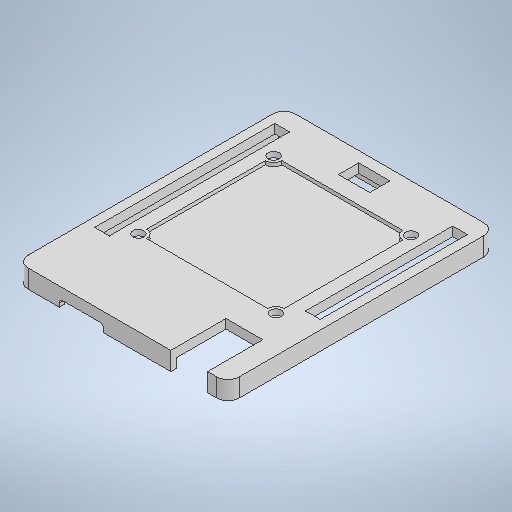
# Autodesk Inventor part: uno_r4_lid
Saved by Autodesk Inventor 2025.2 (Build 292293000, 293)
## iProperties
Created: 2025-03-24
Part Number: uno_r4_lid
Material: Generic
Document SubType Name: Modeling
Designer: caomi
Density: 1 g/cm^3
Appearance: Default
Author: caomi
Autodesk Inventor part; units mm, degrees
ref_plane "YZ Plane" through (0, 0, 0) normal (1, 0, 0) x (0, 1, 0)
ref_plane "XZ Plane" through (0, 0, 0) normal (0, 1, 0) x (-1, 0, 0)
ref_plane "XY Plane" through (0, 0, 0) normal (0, 0, 1) x (1, 0, 0)
sketch "Sketch1" plane through (0, 0, 0) normal (0, 1, 0) x (-1, 0, 0)
  line L0 (0, 0) -> (53.34, 0) construction
  line L1 (53.34, 0) -> (53.34, -68.58) construction
  line L2 (53.34, -68.58) -> (0, -68.58) construction
  line L3 (0, -68.58) -> (0, 0) construction
  line L4 (55.34, -70.58) -> (55.34, 2)
  line L5 (55.34, 2) -> (-2, 2)
  line L6 (-2, 2) -> (-2, -70.58)
  line L7 (-2, -70.58) -> (55.34, -70.58)
  dimension "d0" = 53.34
  dimension "d1" = 68.58
  dimension "d2" = 2
  constraints: 16 end point, 4 parallel, 2 perpendicular, 1 horizontal, 3 other
  measures "d0" distance of L0.start L0.end
  measures "d1" distance of L2.end L0.start
  measures "d2" distance between parallel lines of L1 L4
extrude "Extrusion1" add sketch "Sketch1" against normal blind 5
fillet "Fillet1" radius 3 4 edges at (-55.34, -2.5, 2) (-55.34, -2.5, -70.58) (2, -2.5, -70.58) (2, -2.5, 2)
shell "Shell1" thickness 1.5 removed faces 1 at (-17.1133, -5, -45.3867)
sketch "Sketch2" plane through (0, -5, 0) normal (0, -1, 0) x (1, 0, 0)
  line L0 (-53.34, 0) -> (-53.34, -68.58) construction
  line L1 (-52.34, 0.5) -> (-1, 0.5) projected
  line L2 (-1, 2) -> (-52.34, 2) projected
  line L3 (-43.84, 0.5) -> (-31.84, 0.5)
  line L4 (-31.84, 0.5) -> (-31.84, 2)
  line L5 (-31.84, 2) -> (-43.84, 2)
  line L6 (-43.84, 2) -> (-43.84, 0.5)
  line L7 (-13.54, 2) -> (-3.54, 2)
  line L8 (-3.54, 2) -> (-3.54, -13)
  line L9 (-3.54, -13) -> (-13.54, -13)
  line L10 (-13.54, -13) -> (-13.54, 2)
  dimension "d8" = 12
  dimension "d15" = 9.5
  dimension "d16" = 39.8
  dimension "d17" = 10
  dimension "d18" = 15
  constraints: 16 end point, 4 parallel, 3 point on line, 2 horizontal, 2 perpendicular
  measures "d8" distance between parallel lines of L4 L6
  measures "d15" distance from line of L0 L5.end
  measures "d16" distance between parallel lines of L0 L10
  measures "d17" distance between parallel lines of L8 L10
  measures "d18" distance of L9.end L7.start
extrude "Extrusion2" cut sketch "Sketch2" against normal blind 2 contours L6 L2 L4 L1
fillet "Fillet2" radius 1 2 edges at (-43.84, -3, 1.25) (-31.84, -3, 1.25)
extrude "Extrusion3" cut sketch "Sketch2" against normal through all contours L10 L2 L8 L1 | L1 L8 L9 L10
sketch "Sketch3" plane through (0, 0, 0) normal (0, 1, 0) x (1, 0, 0)
  line L0 (-53.34, 0) -> (-53.34, 68.58) construction
  line L1 (-52.84, 65.58) -> (-48.84, 65.58)
  line L2 (-48.84, 65.58) -> (-48.84, 16.58)
  line L3 (-48.84, 16.58) -> (-52.84, 16.58)
  line L4 (-52.84, 16.58) -> (-52.84, 65.58)
  line L5 (-53.34, 68.58) -> (0, 68.58) construction
  line L6 (-0.5, 65.58) -> (-4.5, 65.58)
  line L7 (-4.5, 65.58) -> (-4.5, 25.58)
  line L8 (-4.5, 25.58) -> (-0.5, 25.58)
  line L9 (-0.5, 25.58) -> (-0.5, 65.58)
  line L10 (0, 68.58) -> (0, 0) construction
  line L11 (-32.14, 67.68) -> (-23.64, 67.68)
  line L12 (-23.64, 67.68) -> (-23.64, 62.18)
  line L13 (-23.64, 62.18) -> (-32.14, 62.18)
  line L14 (-32.14, 62.18) -> (-32.14, 67.68)
  dimension "d19" = 0.5
  dimension "d20" = 4
  dimension "d23" = 3
  dimension "d24" = 52
  dimension "d25" = 0.5
  dimension "d26" = 3
  dimension "d27" = 40
  dimension "d28" = 21.2
  dimension "d29" = 8.5
  dimension "d30" = 5.5
  dimension "d31" = 0.9
  constraints: 24 end point, 6 parallel, 3 horizontal, 3 perpendicular, 1 collinear
  measures "d19" distance between parallel lines of L0 L4
  measures "d20" distance of L2.end L3.end
  measures "d23" distance between parallel lines of L5 L1
  measures "d24" distance between parallel lines of L3 L5
  measures "d25" distance between parallel lines of L10 L9
  measures "d26" distance from line of L5 L6.start
  measures "d27" distance of L8.end L6.start
  measures "d28" distance from line of L0 L11.start
  measures "d29" distance of L11.start L11.end
  measures "d30" distance of L13.end L11.start
  measures "d31" vertical distance of L0.end L11.start
extrude "Extrusion4" cut sketch "Sketch3" against normal blind 5
sketch "Sketch4" plane through (0, 0, 0) normal (0, 1, 0) x (1, 0, 0)
  line L0 (-48.17, 60.8905) -> (-5.17, 60.8905) construction
  line L1 (-5.17, 60.8905) -> (-5.17, 17.8905) construction
  line L2 (-5.17, 17.8905) -> (-48.17, 17.8905) construction
  line L3 (-48.17, 17.8905) -> (-48.17, 60.8905) construction
  line L4 (-48.17, 60.8905) -> (-5.17, 17.8905) construction
  line L5 (-5.17, 60.8905) -> (-48.17, 17.8905) construction
  line L6 (-45.36, 57.7615) -> (-7.98, 57.7615) construction
  line L7 (-7.98, 57.7615) -> (-7.98, 21.0195) construction
  line L8 (-7.98, 21.0195) -> (-45.36, 21.0195) construction
  line L9 (-45.36, 21.0195) -> (-45.36, 57.7615) construction
  line L10 (-45.36, 57.7615) -> (-7.98, 21.0195) construction
  line L11 (-7.98, 57.7615) -> (-45.36, 21.0195) construction
  circle A0 centre (-7.98, 21.0195) radius 1.5
  circle A1 centre (-45.36, 21.0195) radius 1.5
  circle A2 centre (-45.36, 57.7615) radius 1.5
  circle A3 centre (-7.98, 57.7615) radius 1.5
  circle A4 centre (-7.98, 21.0195) radius 2.25
  circle A5 centre (-45.36, 21.0195) radius 2.25
  circle A6 centre (-7.98, 57.7615) radius 2.25
  circle A7 centre (-45.36, 57.7615) radius 2.25
  line L12 (-10.23, 21.0195) -> (-43.11, 21.0195)
  line L13 (-45.36, 23.2695) -> (-45.36, 55.5115)
  line L14 (-43.11, 57.7615) -> (-10.23, 57.7615)
  line L15 (-7.98, 23.2695) -> (-7.98, 55.5115)
  line L16 (-4.5, 65.58) -> (-0.5, 65.58) projected
  line L17 (-48.84, 65.58) -> (-4.5, 65.58) construction
  point P0 (-26.67, 39.3905)
  point P1 (-26.67, 65.58)
  dimension "d34" = 43
  dimension "d35" = 37.38
  dimension "d36" = 36.742
  dimension "d37" = 3
  dimension "d43" = 4.5
  constraints: 34 end point, 8 centre point, 8 coincident, 8 point on circle, 7 point on line, 6 equal radius, 5 midpoint, 4 parallel, 3 collinear, 3 perpendicular, 2 horizontal, 1 vertical alignment
  measures "d34" distance of L1.end L2.end
  measures "d35" distance of L7.end L8.end
  measures "d36" distance of L8.end L6.start
  measures "d37" diameter of A0
  measures "d43" diameter of A4
sketch "Sketch7" plane through (-52.34, -1.5, -69.08) normal (0, -1, 0) x (1, 0, 0)
  line L0 (3.5, 52.5) -> (3.5, 3.5) projected
  line L1 (3.5, 3.5) -> (-0.5, 3.5) projected
  line L2 (-0.5, 3.5) -> (-0.5, 52.5) projected
  line L3 (-0.5, 52.5) -> (3.5, 52.5) projected
  line L4 (47.84, 43.5) -> (51.84, 43.5) projected
  line L5 (51.84, 43.5) -> (51.84, 3.5) projected
  line L6 (51.84, 3.5) -> (47.84, 3.5) projected
  line L7 (47.84, 3.5) -> (47.84, 43.5) projected
  line L8 (28.7, 6.9) -> (28.7, 1.4) projected
  line L9 (28.7, 1.4) -> (20.2, 1.4) projected
  line L10 (20.2, 1.4) -> (20.2, 6.9) projected
  line L11 (20.2, 6.9) -> (28.7, 6.9) projected
  line L12 (48.8, 69.58) -> (48.8, 56.08) projected
  line L13 (48.8, 56.08) -> (38.8, 56.08) projected
  line L14 (38.8, 56.08) -> (38.8, 69.58) projected
  line L15 (0, 69.58) -> (38.8, 69.58) projected
  arc A0 (0, 69.58) -> (-1.5, 68.08) centre (0, 68.08) ccw projected
  line L16 (-1.5, 1.5) -> (-1.5, 68.08) projected
  arc A1 (-1.5, 1.5) -> (0, 0) centre (0, 1.5) ccw projected
  line L17 (51.34, 0) -> (0, 0) projected
  arc A2 (51.34, 0) -> (52.84, 1.5) centre (51.34, 1.5) ccw projected
  line L18 (52.84, 68.08) -> (52.84, 1.5) projected
  arc A3 (52.84, 68.08) -> (51.34, 69.58) centre (51.34, 68.08) ccw projected
  line L19 (48.8, 69.58) -> (51.34, 69.58) projected
  point P0 (52.34, 69.08)
extrude "Extrusion9" add sketch "Sketch7" along normal blind 1
extrude "Extrusion5" cut sketch "Sketch4" against normal through all contours A0 | A1 | A2 | A3
sketch "Sketch5" plane through (-52.34, -1.5, -69.08) normal (0, -1, 0) x (1, 0, 0)
  line L0 (46.9434, 46.2419) -> (43.7934, 44.4232)
  line L1 (43.7934, 44.4232) -> (40.6434, 46.2419)
  line L2 (40.6434, 46.2419) -> (40.6434, 49.8792)
  line L3 (40.6434, 49.8792) -> (43.7934, 51.6978)
  line L4 (43.7934, 51.6978) -> (46.9434, 49.8792)
  line L5 (46.9434, 49.8792) -> (46.9434, 46.2419)
  line L6 (46.9434, 13.1372) -> (46.9434, 9.4999)
  line L7 (46.9434, 9.4999) -> (43.7934, 7.6812)
  line L8 (43.7934, 7.6812) -> (40.6434, 9.4999)
  line L9 (40.6434, 9.4999) -> (40.6434, 13.1372)
  line L10 (40.6434, 13.1372) -> (43.7934, 14.9558)
  line L11 (43.7934, 14.9558) -> (46.9434, 13.1372)
  circle A0 centre (6.98, 48.0605) radius 1.5 projected
  line L12 (10.13, 49.8792) -> (10.13, 46.2419)
  line L13 (10.13, 46.2419) -> (6.98, 44.4232)
  line L14 (6.98, 44.4232) -> (3.83, 46.2419)
  line L15 (3.83, 46.2419) -> (3.83, 49.8792)
  line L16 (3.83, 49.8792) -> (6.98, 51.6978)
  line L17 (6.98, 51.6978) -> (10.13, 49.8792)
  line L18 (9.5634, 13.1372) -> (9.5634, 9.4999)
  line L19 (9.5634, 9.4999) -> (6.4134, 7.6812)
  line L20 (6.4134, 7.6812) -> (3.2634, 9.4999)
  line L21 (3.2634, 9.4999) -> (3.2634, 13.1372)
  line L22 (3.2634, 13.1372) -> (6.4134, 14.9558)
  line L23 (6.4134, 14.9558) -> (9.5634, 13.1372)
  point P0 (43.7934, 48.0605)
  point P1 (43.7934, 48.0605)
  point P2 (43.7934, 11.3185)
  point P3 (43.7934, 11.3185)
  point P4 (6.4134, 11.3185)
  point P5 (6.4134, 11.3185)
  dimension "d40" = 6.3
  constraints: 48 end point, 4 coincident, 4 vertical, 3 equal length, 52 other
  measures "d40" distance between parallel lines of L2 L5
extrude "Extrusion6" cut sketch "Sketch5" along normal up to surface (1 mm away)
extrude "Extrusion7" cut sketch "Sketch4" against normal blind 1 contours A4 L12 A5 L13 A7 L14 A6 L15
equation "\"d2\" = base_wall + tolerance_general"
equation "\"d6\" = base_wall"
equation "\"uno_width\" = 53.34"
equation "\"uno_length\" = 68.58"
equation "\"base_wall\" = 1.5"
equation "\"tolerance_general\" = 0.5"
body "Solid1"
